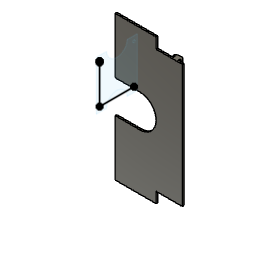
Motor Cover Front (Autodesk Fusion 360 design; units mm, degrees)
Autodesk Fusion 360 part; units mm, degrees
note: some values were not read from the file. Set by a fixed rule: which sketch regions a step uses.
sketch "Sketch1" plane through (0, 0, 0) normal (0, 0, 1) x (1, 0, 0)
  line L0 (0, 0) -> (3.1, 0)
  line L1 (0, 0) -> (-3.1, 0)
  line L2 (3.1, 0) -> (5.4, 0)
  line L3 (-3.1, 0) -> (-5.4, 0)
  line L4 (-5.4, 0) -> (-5.4, 1)
  line L5 (-5.4, 1) -> (-3.0665, 3.3335)
  line L6 (5.4, 0) -> (5.4, 1)
  line L7 (5.4, 1) -> (3.0665, 3.3335)
  line L8 (3.0665, 3.3335) -> (-3.0665, 3.3335)
  line L9 (-3.1, 0) -> (-3.1, -2.1)
  line L10 (3.1, 0) -> (3.1, -2.1)
  line L11 (-1.9, -7.1) -> (-32.5, -7.1)
  arc A0 (-32.5, -7.1) -> (-36.9, -12.1) centre (-32.5, -11.536) ccw
  line L12 (-39.9, -7.1) -> (-39.9, -12.1)
  arc A1 (-34.9, -2.1) -> (-39.9, -7.1) centre (-34.9, -7.1) ccw
  line L13 (-3.1, -2.1) -> (-34.9, -2.1)
  arc A2 (-1.9, -7.1) -> (3.1, -2.1) centre (-1.9, -2.1) ccw
  line L14 (-39.9, -12.1) -> (-39.9, -62.1)
  line L15 (-36.9, -12.1) -> (-36.9, -62.1)
  line L16 (-36.9, -62.1) -> (-39.9, -62.1)
  dimension "d1" = 3.1
  dimension "d2" = 3.1
  dimension "d7" = 2.3
  dimension "d8" = 2.3
  dimension "d9" = 135
  dimension "d10" = 3.3
  dimension "d11" = 135
  dimension "d12" = 3.3
  dimension "d13" = 2.1
  dimension "d14" = 2.1
  dimension "d24" = 31.8
  dimension "d25" = 50
  dimension "d26" = 50
  constraint coincident L0.start L1.start
  constraint horizontal L0
  constraint parallel L0 L1
  constraint parallel L0 L2
  constraint horizontal L3
  constraint perpendicular L3 L4
  constraint perpendicular L2 L6
  constraint perpendicular L6 L8
  constraint perpendicular L3 L9
  constraint perpendicular L2 L10
  constraint horizontal L11
  constraint perpendicular L9 L13
  constraint tangent L10 A2
  constraint tangent L11 A2
  constraint parallel L12 L14
  constraint vertical L15
  constraint perpendicular L14 L16
  measures "d1" distance of L0.start L0.end
  measures "d2" distance of L0.start L1.end
  measures "d7" distance of L0.end L2.end
  measures "d8" distance of L1.end L3.end
  measures "d9" angle of L4 L5
  measures "d10" distance of L4.end L5.end
  measures "d11" angle of L6 L7
  measures "d12" distance of L6.end L7.end
  measures "d13" distance of L1.end L9.end
  measures "d14" distance of L0.end L10.end
  measures "d24" distance of L9.end A1.start
  measures "d25" distance of L12.end L14.end
  measures "d26" distance of A0.end L15.end
extrude "Extrude1" add sketch "Sketch1" along normal blind 60
sketch "Sketch2" plane through (-36.9, 0, 0) normal (1, 0, 0) x (0, 1, 0)
  line L0 (-62.1, 0) -> (-12.1, 0)
  line L1 (-12.1, 0) -> (-12.1, 60)
  line L2 (-12.1, 60) -> (-62.1, 60)
  line L3 (-62.1, 60) -> (-62.1, 0)
  line L4 (-12.1, 60) -> (-62.1, 60)
  line L5 (-62.1, 60) -> (-58.1, 60)
  line L6 (-12.1, 60) -> (-16.1, 60)
  line L7 (-16.1, 60) -> (-58.1, 60)
  line L8 (-58.1, 60) -> (-58.1, 54)
  line L9 (-58.1, 54) -> (-58.1, 6)
  line L10 (-58.1, 6) -> (-16.1, 6)
  line L11 (-16.1, 6) -> (-16.1, 54)
  line L12 (-16.1, 54) -> (-58.1, 54)
  circle A0 centre (-58.1, 54) radius 1.5
  circle A1 centre (-16.1, 54) radius 1.5
  circle A2 centre (-16.1, 6) radius 1.5
  circle A3 centre (-58.1, 6) radius 1.5
  dimension "d29" = 4
  dimension "d30" = 4
  dimension "d31" = 42
  dimension "d32" = 3
  dimension "d33" = 3
  dimension "d34" = 3
  dimension "d35" = 3
  constraint coincident L1.end L2.start
  constraint coincident L2.end L3.start
  constraint perpendicular L3 L5
  constraint perpendicular L1 L6
  constraint perpendicular L2 L8
  constraint perpendicular L2 L9
  constraint perpendicular L9 L10
  constraint perpendicular L10 L11
  constraint perpendicular L9 L12
  constraint coincident L8.end L9.start
  constraint coincident L11.end L12.start
  constraint coincident L10.end L11.start
  constraint coincident L9.end L10.start
  measures "d29" distance of L2.end L5.end
  measures "d30" distance of L1.end L6.end
  measures "d31" distance of L9.end L10.end
  measures "d32" diameter of A0
  measures "d33" diameter of A1
  measures "d34" diameter of A2
  measures "d35" diameter of A3
extrude "Extrude2" cut sketch "Sketch2" against normal blind 30 contours L8 L12 A0 | L8 L9 A0 | L9 L12 A0 | L11 L12 A1 | L11 L12 A1 | L9 L10 A3 | L9 L10 A3 | L10 L11 A2 | L10 L11 A2
sketch "Sketch3" plane through (-36.9, 0, 0) normal (1, 0, 0) x (0, 1, 0)
  circle A0 centre (-58.1, 6) radius 1.5
  circle A1 centre (-58.1, 54) radius 1.5
  circle A2 centre (-16.1, 6) radius 1.5
  circle A3 centre (-16.1, 54) radius 1.5
  line L0 (-62.1, 0) -> (-12.1, 0)
  line L1 (-12.1, 0) -> (-12.1, 60)
  line L2 (-12.1, 60) -> (-62.1, 60)
  line L3 (-62.1, 60) -> (-62.1, 0)
  line L4 (-62.1, 0) -> (-37.1, 0)
  line L5 (-37.1, 0) -> (-37.1, 60)
  circle A4 centre (-37.1, 60) radius 12.5
  circle A5 centre (-37.1, 0) radius 12.5
  dimension "d38" = 25
  dimension "d39" = 25
  dimension "d40" = 25
  constraint coincident L0.start L3.end
  constraint perpendicular L1 L4
  constraint midpoint L2 L5.end
  constraint coincident L5.end A4.centre
  constraint coincident L4.end L5.start
  measures "d38" distance of L0.start L4.end
  measures "d39" diameter of A4
  measures "d40" diameter of A5
extrude "Extrude3" cut sketch "Sketch3" against normal blind 3 contours L0 L5 A5 | L0 L4 L5 A5 | L2 L5 A4 | L2 L5 A4
sketch "Sketch4" plane through (-36.9, 0, 0) normal (1, 0, 0) x (0, 1, 0)
  arc A0 (-24.6, 0) -> (-49.6, 0) centre (-37.1, 0) ccw
  line L0 (-24.6, 0) -> (-12.1, 0)
  line L1 (-12.1, 0) -> (-12.1, 60)
  line L2 (-12.1, 60) -> (-24.6, 60)
  arc A1 (-49.6, 60) -> (-24.6, 60) centre (-37.1, 60) ccw
  line L3 (-49.6, 60) -> (-62.1, 60)
  line L4 (-62.1, 60) -> (-62.1, 0)
  line L5 (-62.1, 0) -> (-49.6, 0)
  circle A2 centre (-58.1, 6) radius 1.5
  circle A3 centre (-58.1, 54) radius 1.5
  circle A4 centre (-16.1, 6) radius 1.5
  circle A5 centre (-16.1, 54) radius 1.5
  line L6 (-58.1, 54) -> (-58.1, 6)
  line L7 (-58.1, 6) -> (-16.1, 6)
  line L8 (-58.1, 54) -> (-58.1, 52.5)
  constraint coincident A3.centre L6.start
  constraint coincident A2.centre L6.end
  constraint coincident A4.centre L7.end
  constraint coincident A3 L8.end
  constraint coincident L6 L8.end
extrude "Extrude4" cut 1 faces at (-37.9, -62.1, 20) along direction (0, 1, 0) blind 51
sketch "Sketch5" plane through (0, -7.1, 0) normal (0, -1, 0) x (1, 0, 0)
  line L0 (-32.5, 0) -> (-1.9, 0)
  line L1 (-1.9, 0) -> (-1.9, 60)
  line L2 (-1.9, 60) -> (-32.5, 60)
  line L3 (-32.5, 60) -> (-32.5, 0)
  line L4 (-32.5, 0) -> (-40, 0)
  line L5 (-40, 0) -> (-40, 60)
  line L6 (-40, 60) -> (-32.5, 60)
  line L7 (-32.5, 60) -> (-32.5, 0)
  line L8 (-40, 0) -> (-30, 0)
  line L9 (-30, 0) -> (-30, 60)
  line L10 (-30, 60) -> (-40, 60)
  line L11 (-40, 0) -> (-40, 60)
  line L12 (-40, 60) -> (-30, 60)
  constraint coincident L0.start L3.end
  constraint perpendicular L3 L4
  constraint perpendicular L4 L5
  constraint coincident L2.end L3.start
  constraint coincident L0 L8.end
  constraint perpendicular L5 L8
  constraint coincident L2 L9.end
  constraint perpendicular L2 L9
extrude "Extrude6" cut 1 faces at (-39.9, -8.4333, 20) along direction (1, 0, 0) blind 8
sketch "Sketch6" plane through (0, -7.1, 0) normal (0, -1, 0) x (1, 0, 0)
  line L0 (-39.9, 0) -> (-1.9, 0)
  line L1 (-1.9, 0) -> (-1.9, 60)
  line L2 (-1.9, 60) -> (-39.9, 60)
  line L3 (-39.9, 60) -> (-39.9, 0)
  line L4 (-39.9, 0) -> (-30, 0)
  line L5 (-30, 0) -> (-30, 60)
  line L6 (-30, 60) -> (-39.9, 60)
  line L7 (-39.9, 60) -> (-39.9, 0)
  constraint coincident L0.start L3.end
  constraint coincident L0 L4.end
  constraint perpendicular L3 L4
  constraint coincident L2 L5.end
  constraint perpendicular L2 L5
  constraint coincident L2.end L3.start
  constraint perpendicular L3 L6
extrude "Extrude7" cut sketch "Sketch6" against normal blind 10 contours L0 L2 L3 L4 L5 L6 L7
extrude "Extrude8" cut 1 faces at (-11.2667, -7.1, 20) along direction (0, 1, 0) blind 3
extrude "Extrude9" cut 1 faces at (-1.9, -6.1, 20) along direction (1, 0, 0) blind 5
fillet "Fillet1" radius 3 1 edges at (2.6826, -4.1, 30)
sketch "Sketch7" plane through (0, 0, 0) normal (0, 0, -1) x (1, 0, 0)
  arc A0 (3.1, 1.1) -> (0.1, 4.1) centre (0.1, 1.1) ccw
  line L0 (0.1, 4.1) -> (-30, 4.1)
  line L1 (-30, 4.1) -> (-30, 2.1)
  line L2 (-30, 2.1) -> (-3.1, 2.1)
  line L3 (-3.1, 2.1) -> (-3.1, 0)
  line L4 (-3.1, 0) -> (-5.4, 0)
  line L5 (-5.4, 0) -> (-5.4, -1)
  line L6 (-5.4, -1) -> (-3.0665, -3.3335)
  line L7 (-3.0665, -3.3335) -> (3.0665, -3.3335)
  line L8 (3.0665, -3.3335) -> (5.4, -1)
  line L9 (5.4, -1) -> (5.4, 0)
  line L10 (5.4, 0) -> (3.1, 0)
  line L11 (3.1, 0) -> (3.1, 1.1)
  line L12 (-3.4865, 4.1) -> (6, 4.1)
  line L13 (3.1, 0) -> (3.1, 4.1)
  constraint coincident L0 L12.start
  constraint coincident L10.end L11.start
  constraint coincident L12 L13.end
  constraint perpendicular L12 L13
extrude "Extrude10" add sketch "Sketch7" against normal blind 60 contours A0 L12 L13
extrude "Extrude11" cut 1 faces at (-30, -3.4333, 20) along direction (1, 0, 0) blind 0.1
extrude "Extrude12" add 1 faces at (-29.9, -3.4333, 20) along direction (-1, 0, 0) blind 49
extrude "Extrude13" add 1 faces at (1.0333, -2.0667, 0) along direction (0, 0, -1) blind 116
sketch "Sketch8" plane through (0, 0, -116) normal (0, 0, -1) x (1, 0, 0)
  line L0 (-78.9, 2.1) -> (-3.1, 2.1)
  line L1 (-3.1, 2.1) -> (-3.1, 0)
  line L2 (-3.1, 0) -> (-5.4, 0)
  line L3 (-5.4, 0) -> (-5.4, -1)
  line L4 (-5.4, -1) -> (-3.0665, -3.3335)
  line L5 (-3.0665, -3.3335) -> (3.0665, -3.3335)
  line L6 (3.0665, -3.3335) -> (5.4, -1)
  line L7 (5.4, -1) -> (5.4, 0)
  line L8 (5.4, 0) -> (3.1, 0)
  line L9 (3.1, 0) -> (3.1, 4.1)
  line L10 (3.1, 4.1) -> (-78.9, 4.1)
  line L11 (-78.9, 4.1) -> (-78.9, 2.1)
  line L12 (0, 0) -> (10, 0)
  line L13 (10, 0) -> (10, 4.1)
  line L14 (0, 0) -> (-10, 0)
  line L15 (-10, 0) -> (-10, 4.1)
  line L16 (0, 0) -> (-22, 0)
  line L17 (-22, 0) -> (-22, 2.1)
  line L18 (-3.1, 2.1) -> (-3.1, 4.1)
  line L19 (-3.1, 4.1) -> (-22, 4.1)
  line L20 (-22, 4.1) -> (-22, 2.1)
  line L21 (-10, 0) -> (-10, -5)
  line L22 (-10, -5) -> (7.5, -5)
  line L23 (7.5, 4) -> (-10, 4.1)
  line L24 (7.5, 4) -> (7.5, -5)
  dimension "d65" = 4.1
  dimension "d66" = 2
  constraint coincident L12.start L14.start
  constraint perpendicular L9 L12
  constraint perpendicular L12 L13
  constraint perpendicular L3 L14
  constraint coincident L10 L15.end
  constraint perpendicular L10 L15
  constraint perpendicular L9 L16
  constraint coincident L0 L17.end
  constraint perpendicular L0 L17
  constraint coincident L0.end L1.start
  constraint perpendicular L10 L18
  constraint coincident L10 L19.end
  constraint perpendicular L18 L19
  constraint perpendicular L0 L20
  constraint perpendicular L16 L21
  constraint perpendicular L21 L22
  constraint perpendicular L22 L24
  measures "d65" distance of L12.end L13.end
  measures "d66" distance of L0.end L18.end
extrude "Extrude14" cut sketch "Sketch8" against normal blind 13 contours L0 L10 L15 L19 L20 | L0 L15 L16 L17 | L0 L15 L18 L23 | L0 L1 L2 L14 L15 L16 | L1 L9 L12 L14 L16 L18 L23 | L3 L4 L5 L6 L7 L12 L14 L16 L21 L22 L24 | L2 L3 L4 L5 L6 L7 L8 L12 L14 L16 | L8 L9 L12 L23 L24
sketch "Sketch9" plane through (0, -4.1, 0) normal (0, -1, 0) x (1, 0, 0)
  line L0 (-22, -116) -> (-22, -103)
  line L1 (-22, -103) -> (-10, -103)
  line L2 (-10, -103) -> (-10, -116)
  line L3 (-10, -116) -> (3.1, -116)
  line L4 (3.1, -116) -> (3.1, 60)
  line L5 (3.1, 60) -> (-78.9, 60)
  line L6 (-78.9, 60) -> (-78.9, -116)
  line L7 (-78.9, -116) -> (-22, -116)
  line L8 (-10, -103) -> (3.1, -103)
  line L9 (3.1, -103) -> (3.1, -116)
  line L10 (3.1, -116) -> (-10, -116)
  line L11 (-10, -116) -> (-10, -103)
  constraint coincident L1.end L2.start
  constraint coincident L4 L8.end
  constraint perpendicular L4 L8
  constraint coincident L3.end L4.start
  constraint coincident L2.end L3.start
extrude "Extrude15" cut sketch "Sketch9" against normal blind 4 contours L2 L3 L4 L8 L9 L10 L11
sketch "Sketch10" plane through (0, 0, 60) normal (0, 0, 1) x (-1, 0, 0)
  line L0 (78.9, 4.1) -> (-3.1, 4.1)
  line L1 (-3.1, 4.1) -> (-3.1, 0)
  line L2 (-3.1, 0) -> (-5.4, 0)
  line L3 (-5.4, 0) -> (-5.4, -1)
  line L4 (-5.4, -1) -> (-3.0665, -3.3335)
  line L5 (-3.0665, -3.3335) -> (3.0665, -3.3335)
  line L6 (3.0665, -3.3335) -> (5.4, -1)
  line L7 (5.4, -1) -> (5.4, 0)
  line L8 (5.4, 0) -> (3.1, 0)
  line L9 (3.1, 0) -> (3.1, 2.1)
  line L10 (3.1, 2.1) -> (78.9, 2.1)
  line L11 (78.9, 2.1) -> (78.9, 4.1)
  line L12 (0, 4.1) -> (-10, 4.1)
  line L13 (0, 4.1) -> (22, 4.1)
  line L14 (22, 4.1) -> (22, -7)
  line L15 (22, -7) -> (-10, -7)
  line L16 (-10, -7) -> (-10, 4.1)
  constraint coincident L0 L12.start
  constraint perpendicular L9 L12
  constraint coincident L0 L13.end
  constraint parallel L0 L13
  constraint perpendicular L13 L14
  constraint perpendicular L14 L15
  constraint perpendicular L12 L16
extrude "Extrude16" cut sketch "Sketch10" against normal blind 13 contours L0 L1 L2 L3 L4 L5 L6 L7 L8 L9 L10 L12 L13 L14 | L1 L2 L3 L4 L5 L6 L7 L8 L9 L10 L12 L14 L15 L16
sketch "Sketch11" plane through (0, 0, -103) normal (0, 0, -1) x (1, 0, 0)
  line L0 (3.1, 4.1) -> (-22, 4.1)
  line L1 (-22, 4.1) -> (-22, 2.1)
  line L2 (-22, 2.1) -> (-3.1, 2.1)
  line L3 (-3.1, 2.1) -> (-3.1, 0)
  line L4 (-3.1, 0) -> (-5.4, 0)
  line L5 (-5.4, 0) -> (-5.4, -1)
  line L6 (-5.4, -1) -> (-3.0665, -3.3335)
  line L7 (-3.0665, -3.3335) -> (3.0665, -3.3335)
  line L8 (3.0665, -3.3335) -> (5.4, -1)
  line L9 (5.4, -1) -> (5.4, 0)
  line L10 (5.4, 0) -> (3.1, 0)
  line L11 (3.1, 0) -> (3.1, 4.1)
  line L12 (0, 0) -> (0, 4.1)
  line L13 (0, 4.1) -> (3.1, 4.1)
  line L14 (0, 4.1) -> (10, 4.1)
  line L15 (10, 4.1) -> (3.1, 4.1)
  line L16 (10, 4.1) -> (10, 2.1)
  line L17 (10, 2.1) -> (3.1, 2.1)
  line L18 (3.1, 2.1) -> (3.1, 4.1)
  dimension "d73" = 2
  constraint coincident L12.start origin
  constraint coincident L0 L12.end
  constraint perpendicular L0 L12
  constraint coincident L0.start L11.end
  constraint perpendicular L12 L14
  constraint perpendicular L11 L15
  constraint perpendicular L14 L16
  constraint coincident L11 L17.end
  constraint perpendicular L11 L17
  measures "d73" distance of L14.end L16.end
extrude "Extrude17" add sketch "Sketch11" against normal blind 150 contours L11 L14 L15 L16 L17 L18
extrude "Extrude18" cut 1 faces at (-78.9, -2.7667, -57.3333) along direction (1, 0, 0) blind 6.9
sketch "Sketch12" plane through (0, -4.1, 0) normal (0, -1, 0) x (1, 0, 0)
  line L0 (-72, 60) -> (-72, -116)
  line L1 (-72, -116) -> (-22, -116)
  line L2 (-22, -116) -> (-22, -103)
  line L3 (-22, -103) -> (10, -103)
  line L4 (10, -103) -> (10, 47)
  line L5 (10, 47) -> (-22, 47)
  line L6 (-22, 47) -> (-22, 60)
  line L7 (-22, 60) -> (-72, 60)
  line L8 (10, 47) -> (10, -103)
  line L9 (10, -103) -> (10, -28)
  line L10 (10, -28) -> (-22, -28)
  line L11 (-22, -28) -> (-22, -8)
  line L12 (-22, -8) -> (-72, -8)
  line L13 (-72, -8) -> (-72, -48)
  line L14 (-72, -48) -> (-22, -48)
  line L15 (-22, -48) -> (-22, -28)
  constraint coincident L4.end L5.start
  constraint coincident L3.end L4.start
  constraint midpoint L8 L9.end
  constraint perpendicular L9 L10
  constraint perpendicular L5 L11
  constraint coincident L0 L12.end
  constraint perpendicular L0 L12
  constraint coincident L0 L13.end
  constraint perpendicular L13 L14
  constraint perpendicular L14 L15
extrude "Extrude19" cut sketch "Sketch12" against normal blind 5 contours L0 L11 L12 L13 L14 L15
fillet "Fillet2" radius 20 1 edges at (-22, -3.1, -48)
fillet "Fillet3" radius 20 1 edges at (-22, -3.1, -8)
